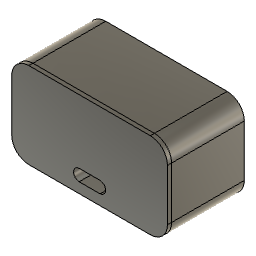
LD2410B Enclosure (Autodesk Fusion 360 design; units mm, degrees)
Autodesk Fusion 360 part; units mm, degrees
sketch "Sketch1" plane through (0, 0, 0) normal (0, 1, 0) x (1, 0, 0)
  line L0 (0, 25.4245) -> (0, -84.4349) construction
  line L1 (0, -3) -> (-3.0467, -3)
  line L2 (-2.98, -4.7) -> (1.5261, -4.7) construction
  arc A0 (-3.0467, -3) -> (-2.98, -6.4013) centre (-2.98, -4.7) ccw
  line L3 (-2.98, -6.4013) -> (0, -6.4013)
  line L4 (2.98, -6.4013) -> (0, -6.4013)
  arc A1 (2.98, -6.4013) -> (3.0467, -3) centre (2.98, -4.7) ccw
  line L5 (0, -3) -> (3.0467, -3)
  line L6 (0, 0) -> (-17.7, 0)
  line L7 (-22.7, -5) -> (-22.7, -20)
  line L8 (-17.7, -25) -> (0, -25)
  line L9 (0, -20) -> (-17.7, -20)
  line L10 (-17.7, -20) -> (-17.7, -12.6)
  line L11 (-17.7, -12.6) -> (0, -12.6)
  line L12 (17.7, -25) -> (0, -25)
  line L13 (0, -20) -> (17.7, -20)
  line L14 (17.7, -20) -> (17.7, -12.6)
  line L15 (22.7, -5) -> (22.7, -20)
  line L16 (17.7, -12.6) -> (0, -12.6)
  line L17 (0, 0) -> (17.7, 0)
  line L18 (17.7, -23.8) -> (-17.7, -23.8)
  line L19 (-21.5, -20) -> (-21.5, -5)
  line L20 (-17.7, -1.2) -> (17.7, -1.2)
  line L21 (21.5, -5) -> (21.5, -20)
  line L22 (-17.7, -20) -> (-17.7, -22)
  line L23 (-17.7, -22) -> (17.7, -22)
  line L24 (17.7, -22) -> (17.7, -20)
  line L25 (17.7, -12.6) -> (17.7, -10.6)
  line L26 (17.7, -10.6) -> (-17.7, -10.6)
  line L27 (-17.7, -10.6) -> (-17.7, -12.6)
  circle A2 centre (-18.3, -9.2) radius 3
  circle A3 centre (-18.3, -9.2) radius 1.4
  circle A4 centre (18.3, -9.2) radius 1.4
  circle A5 centre (18.3, -9.2) radius 3
  arc A6 (17.7, -23.8) -> (21.5, -20) centre (17.7, -20) ccw
  arc A7 (17.7, -25) -> (22.7, -20) centre (17.7, -20) ccw
  arc A8 (21.5, -5) -> (17.7, -1.2) centre (17.7, -5) ccw
  arc A9 (22.7, -5) -> (17.7, 0) centre (17.7, -5) ccw
  arc A10 (-21.5, -20) -> (-17.7, -23.8) centre (-17.7, -20) ccw
  arc A11 (-22.7, -20) -> (-17.7, -25) centre (-17.7, -20) ccw
  arc A12 (-17.7, -1.2) -> (-21.5, -5) centre (-17.7, -5) ccw
  arc A13 (-17.7, 0) -> (-22.7, -5) centre (-17.7, -5) ccw
  point P0 (-22.7, 0)
  point P1 (-22.7, -25)
  dimension "d2" = 1.7
  dimension "d3" = 3
  dimension "d4" = 7.4
  dimension "d5" = 17.7
  dimension "d6" = 5
  dimension "d7" = 25
  dimension "d8" = 5
  dimension "d10" = 1.2
  dimension "d12" = 1.2
  dimension "d13" = 1.2
  dimension "d14" = 1.2
  dimension "d15" = 2
  dimension "d16" = 2
  dimension "d28" = 6
  dimension "d29" = 3.2
  dimension "d30" = 2.8
  dimension "d31" = 8
  dimension "d61" = 3.8
  dimension "d62" = 5
  dimension "d63" = 3.8
  dimension "d64" = 5
  dimension "d65" = 3.8
  dimension "d66" = 5
  dimension "d67" = 3.8
  dimension "d68" = 5
  dimension "d71" = 2.98
  constraint coincident L0 L1.start
  constraint perpendicular L0 L1
  constraint parallel L1 L2
  constraint coincident L2.start A0.centre
  constraint coincident L0 L3.end
  constraint tangent A0 L3
  constraint perpendicular L0 L3
  constraint coincident L6.start L0
  constraint symmetric L0 L1.start L5.start
  constraint symmetric L0 L1.end A1.end
  constraint symmetric L0 A0.end L4.start
  constraint symmetric L0 A0 A1
  constraint symmetric L0 L3.end L4.end
  constraint coincident L6.start L17.start
  constraint perpendicular L0 L6
  constraint perpendicular L6 L7
  constraint coincident L0 L8.end
  constraint perpendicular L0 L8
  constraint coincident L0 L9.start
  constraint perpendicular L0 L9
  constraint perpendicular L9 L10
  constraint coincident L0 L11.end
  constraint perpendicular L0 L11
  constraint symmetric L0 L6.start L17.start
  constraint symmetric L0 L8.end L12.end
  constraint symmetric L0 L9.start L13.start
  constraint symmetric L0 L9.end L13.end
  constraint symmetric L0 L10.end L14.end
  constraint symmetric L0 L11.end L16.end
  constraint perpendicular L0 L18
  constraint perpendicular L18 L19
  constraint perpendicular L15 L20
  constraint perpendicular L18 L21
  constraint perpendicular L9 L22
  constraint perpendicular L14 L23
  constraint perpendicular L13 L24
  constraint perpendicular L16 L25
  constraint perpendicular L10 L26
  constraint perpendicular L11 L27
  constraint concentric A2 A3
  constraint symmetric L0 A2 A5
  constraint symmetric L0 A3 A4
  constraint tangent L21 A6
  constraint tangent L18 A6
  constraint tangent L12 A7
  constraint tangent L15 A7
  constraint tangent L21 A8
  constraint tangent L20 A8
  constraint tangent L15 A9
  constraint tangent L17 A9
  constraint tangent L18 A10
  constraint tangent L19 A10
  constraint coincident P1 L8
  constraint coincident P1 L7
  constraint tangent L8 A11
  constraint tangent L7 A11
  constraint tangent L20 A12
  constraint tangent L19 A12
  constraint coincident P0 L6
  constraint coincident P0 L7
  constraint tangent L6 A13
  constraint tangent L7 A13
  measures "d2" distance of L1 L2
  measures "d3" distance of L5 L6
  measures "d4" distance of L9.end L10.end
  measures "d5" distance of L9.start L9.end
  measures "d6" distance of L8 L9
  measures "d7" distance of P0 P1
  measures "d8" distance of L7 L10
  measures "d10" distance of L12 L18
  measures "d12" distance of L15 L21
  measures "d13" distance of L17 L20
  measures "d14" distance of L7 L19
  measures "d16" distance of L14.end L25.end
  measures "d28" diameter of A2
  measures "d29" distance of L19 A2.centre
  measures "d30" diameter of A3
  measures "d31" distance of L20 A2.centre
  measures "d61" radius of A6
  measures "d62" radius of A7
  measures "d63" radius of A8
  measures "d64" radius of A9
  measures "d65" radius of A10
  measures "d66" radius of A11
  measures "d67" radius of A12
  measures "d68" radius of A13
  measures "d71" distance of L0 L2.start
extrude "Extrude1" add sketch "Sketch1" along normal blind 1.2 contours L1 A0 L3 L4 A1 L5 | L6 L7 L8 L12 L15 L17 A7 A9 A11 A13 | L9 L13 L22 L23 L24 | L9 L10 L11 L13 L14 L16 | L11 L16 L25 L26 L27 A2 A5 | L26 L27 A2 | L26 L27 A2 | L25 L26 A5 | L25 L26 A5 | L18 L19 L20 L21 A6 A8 A10 A12 | A3 | A4 makes body 1
extrude "Extrude2" add sketch "Sketch1" against normal blind 3 contours L9 L13 L22 L23 L24 | L11 L16 L25 L26 L27 A2 A5 | L26 L27 A2 | L25 L26 A5 picked at (-17.2824, -11.486) picked at (17.2824, -11.486) bodies 1
extrude "Extrude3" add sketch "Sketch1" against normal blind 20 contours L6 L7 L8 L12 L15 L17 A7 A9 A11 A13 bodies 1
sketch "Sketch2" plane through (0, -20, 0) normal (0, -1, 0) x (1, 0, 0)
  line L0 (17.7, 1.2) -> (-17.7, 1.2)
  line L1 (-21.5, 5) -> (-21.5, 20)
  line L2 (-17.7, 23.8) -> (17.7, 23.8)
  line L3 (21.5, 20) -> (21.5, 5)
  line L4 (-22.7, 20) -> (-22.7, 5)
  line L5 (-17.7, 0) -> (17.7, 0)
  line L6 (22.7, 5) -> (22.7, 20)
  line L7 (17.7, 25) -> (-17.7, 25)
  line L8 (-2.98, 6.4013) -> (0, 6.4013)
  arc A0 (-2.98, 6.4013) -> (-3.0467, 3) centre (-2.98, 4.7) ccw
  line L9 (0, 3) -> (-3.0467, 3)
  line L10 (0, 3) -> (3.0467, 3)
  arc A1 (3.0467, 3) -> (2.98, 6.4013) centre (2.98, 4.7) ccw
  line L11 (2.98, 6.4013) -> (0, 6.4013)
  line L12 (2.98, 7.6013) -> (0, 7.6013)
  line L13 (-2.98, 7.6013) -> (0, 7.6013)
  arc A2 (-2.98, 7.6013) -> (-3.0672, 1.8) centre (-2.98, 4.7) ccw
  line L14 (0, 1.8) -> (-3.0672, 1.8)
  line L15 (0, 1.8) -> (3.0672, 1.8)
  arc A3 (3.0672, 1.8) -> (2.98, 7.6013) centre (2.98, 4.7) ccw
  line L16 (-17.7, 25) -> (0, 25)
  line L17 (17.7, 25) -> (0, 25)
  line L18 (22.7, 5) -> (22.7, 20)
  line L19 (0, 0) -> (17.7, 0)
  line L20 (0, 0) -> (-17.7, 0)
  line L21 (-22.7, 5) -> (-22.7, 20)
  line L22 (0, 23.6) -> (-17.5, 23.6)
  line L23 (-17.5, 23.6) -> (-17.5, 22.4)
  line L24 (-17.5, 22.4) -> (0, 22.4)
  line L25 (-21.3, 19.8) -> (-20.1, 19.8)
  line L26 (-20.1, 19.8) -> (-20.1, 5.2)
  line L27 (-21.3, 19.8) -> (-21.3, 5.2)
  line L28 (-21.3, 5.2) -> (-20.1, 5.2)
  line L29 (-17.5, 1.4) -> (-17.5, 2.6)
  line L30 (-17.5, 2.6) -> (-7.5, 2.6)
  line L31 (-7.5, 2.6) -> (-7.5, 1.4)
  line L32 (-7.5, 1.4) -> (-17.5, 1.4)
  line L33 (0, -25.4245) -> (0, 84.4349)
  line L34 (0, 23.6) -> (17.5, 23.6)
  line L35 (17.5, 22.4) -> (0, 22.4)
  line L36 (17.5, 23.6) -> (17.5, 22.4)
  line L37 (21.3, 19.8) -> (20.1, 19.8)
  line L38 (20.1, 19.8) -> (20.1, 5.2)
  line L39 (21.3, 19.8) -> (21.3, 5.2)
  line L40 (21.3, 5.2) -> (20.1, 5.2)
  line L41 (17.5, 1.4) -> (17.5, 2.6)
  line L42 (17.5, 2.6) -> (7.5, 2.6)
  line L43 (7.5, 1.4) -> (17.5, 1.4)
  line L44 (7.5, 2.6) -> (7.5, 1.4)
  arc A4 (17.7, 1.2) -> (21.5, 5) centre (17.7, 5) ccw
  arc A5 (-21.5, 5) -> (-17.7, 1.2) centre (-17.7, 5) ccw
  arc A6 (-17.7, 23.8) -> (-21.5, 20) centre (-17.7, 20) ccw
  arc A7 (21.5, 20) -> (17.7, 23.8) centre (17.7, 20) ccw
  arc A8 (17.7, 0) -> (22.7, 5) centre (17.7, 5) ccw
  arc A9 (22.7, 20) -> (17.7, 25) centre (17.7, 20) ccw
  arc A10 (-17.7, 25) -> (-22.7, 20) centre (-17.7, 20) ccw
  arc A11 (-22.7, 5) -> (-17.7, 0) centre (-17.7, 5) ccw
  dimension "d23" = 1.2
  dimension "d34" = 1.2
  dimension "d35" = 1.2
  dimension "d36" = 1.2
  dimension "d37" = 0.2
  dimension "d38" = 0.2
  dimension "d39" = 0.2
  dimension "d40" = 4
  dimension "d41" = 4
  dimension "d42" = 4
  dimension "d43" = 4
  dimension "d44" = 7.5
  constraint parallel L2 L22
  constraint perpendicular L22 L23
  constraint perpendicular L23 L24
  constraint perpendicular L1 L25
  constraint perpendicular L0 L26
  constraint perpendicular L0 L27
  constraint perpendicular L26 L28
  constraint perpendicular L24 L29
  constraint perpendicular L29 L30
  constraint perpendicular L30 L31
  constraint perpendicular L29 L32
  constraint symmetric L22.start L33 L34.start
  constraint symmetric L22.end L33 L34.end
  constraint symmetric L23.end L33 L35.start
  constraint symmetric L24.end L33 L35.end
  constraint symmetric L25.start L33 L37.start
  constraint symmetric L25.end L33 L37.end
  constraint symmetric L26.end L33 L38.end
  constraint symmetric L27.end L33 L39.end
  constraint symmetric L29.start L33 L41.start
  constraint symmetric L29.end L33 L41.end
  constraint symmetric L30.end L33 L42.end
  constraint symmetric L31.end L33 L43.start
  measures "d34" distance of L25.start L25.end
  measures "d35" distance of L22 L24
  measures "d36" distance of L29.start L29.end
  measures "d37" distance of L2 L22
  measures "d38" distance of L1 L27
  measures "d39" distance of L0 L32
  measures "d40" distance of L1 L23
  measures "d41" distance of L2 L25
  measures "d42" distance of L0 L28
  measures "d43" distance of L1 L29.end
  measures "d44" distance of L31 L33
extrude "Extrude4" add sketch "Sketch2" along normal blind 1.2 separate body contours L0 L2 L3 L5 L6 L7 L17 L18 L19 L33 A4 A7 A8 A9 | L0 L2 L3 L12 L15 A3 L33 L34 L35 L36 A4 A7 | L0 L1 L2 L4 L5 L7 L16 L20 L21 L33 A5 A6 A10 A11 | L0 L1 L2 L13 A2 L14 L22 L23 L24 L33 A5 A6 | L10 A1 L11 L12 L15 A3 L33 | L8 A0 L9 L13 A2 L14 L33 | L22 L23 L24 L33 | L33 L34 L35 L36 | L25 L26 L27 L28 | L29 L30 L31 L32 | L37 L38 L39 L40 | L41 L42 L43 L44 makes body 2
extrude "Extrude5" add sketch "Sketch2" against normal blind 8 contours L10 A1 L11 L12 L15 A3 L33 | L8 A0 L9 L13 A2 L14 L33 bodies 2
extrude "Extrude7" add sketch "Sketch2" against normal blind 2.5 contours L22 L23 L24 L33 | L33 L34 L35 L36 | L25 L26 L27 L28 | L29 L30 L31 L32 | L37 L38 L39 L40 | L41 L42 L43 L44 bodies 2
sketch "Sketch4" plane through (17.5, 0, 0) normal (1, 0, 0) x (0, 1, 0)
  line L0 (-20, 23.6) -> (-20, 22.4)
  line L1 (-20, 22.4) -> (-17.5, 22.4)
  line L2 (-17.5, 22.4) -> (-17.5, 23.6)
  line L3 (-17.5, 23.6) -> (-20, 23.6)
  line L4 (-19, 24.1) -> (-18.5, 23.6)
  line L5 (-19, 24.1) -> (-17.815, 24.1) construction
  line L6 (-19, 24.1) -> (-19.5, 23.6)
  line L7 (-18.5, 23.6) -> (-19.5, 23.6)
  line L8 (-17.5, 5.2) -> (-17.5, 19.8) construction
  line L9 (-17.5, 12.5) -> (-15.1425, 12.5) construction
  line L10 (-18.5, 1.4) -> (-19.5, 1.4)
  line L11 (-19, 0.9) -> (-19.5, 1.4)
  line L12 (-19, 0.9) -> (-18.5, 1.4)
  line L13 (-18.2586, 23.5) -> (-19.7414, 23.5)
  line L14 (-19, 24.2414) -> (-19.7414, 23.5)
  line L15 (-19, 24.2414) -> (-18.2586, 23.5)
  line L16 (-19, 0.7586) -> (-19.7414, 1.5)
  line L17 (-19, 0.7586) -> (-18.2586, 1.5)
  line L18 (-18.2586, 1.5) -> (-19.7414, 1.5)
  dimension "d47" = 45
  dimension "d48" = 0.5
  dimension "d49" = 1
  dimension "d57" = 0.1
  constraint horizontal L5
  constraint coincident L3 L4.end
  constraint coincident L3 L6.end
  constraint perpendicular L4 L6
  constraint midpoint L8 L9.start
  constraint perpendicular L8 L9
  constraint symmetric L4.start L9 L11.start
  constraint symmetric L4.end L9 L10.start
  constraint symmetric L6.end L9 L10.end
  constraint symmetric L9 L13.start L17.end
  constraint symmetric L9 L13.end L16.end
  constraint symmetric L9 L14.start L16.start
  measures "d47" angle of L4 L5
  measures "d48" distance of L3 L4.start
  measures "d49" distance of L2 L4.end
extrude "Extrude8" add sketch "Sketch4" against normal up to surface (35 mm away) contours L3 L4 L6 L7 bodies 2
extrude "Extrude9" add sketch "Sketch4" against normal up to surface (10 mm away) contours L10 L11 L12 bodies 2
extrude "Extrude10" add sketch "Sketch4" against normal up to surface (9 mm away) from surface at -26 contours L10 L11 L12 bodies 2
extrude "Extrude11" cut sketch "Sketch4" against normal blind 35.6 from surface at 0.3 contours L3 L4 L6 L14 L15 | L10 L11 L12 bodies 1
sketch "Sketch5" plane through (0, 1.2, 0) normal (0, 1, 0) x (-1, 0, 0)
  line L0 (-17.7, 0) -> (17.7, 0)
  arc A0 (17.7, 0) -> (22.7, 5) centre (17.7, 5) ccw
  line L1 (22.7, 5) -> (22.7, 20)
  arc A1 (22.7, 20) -> (17.7, 25) centre (17.7, 20) ccw
  line L2 (17.7, 25) -> (-17.7, 25)
  arc A2 (-17.7, 25) -> (-22.7, 20) centre (-17.7, 20) ccw
  line L3 (-22.7, 20) -> (-22.7, 5)
  arc A3 (-22.7, 5) -> (-17.7, 0) centre (-17.7, 5) ccw
  line L4 (22.7, 12.5) -> (-22.7, 12.5) construction
  line L5 (0, 25) -> (0, 0) construction
  spline S0 degree 2 poles (0.0295, 1.603) (-2.2457, 1.603) (-4.2468, 2.4665) knots 0 0 0 1 1 1
  spline S1 degree 2 poles (-4.2468, 2.4665) (-6.2478, 3.33) (-7.7281, 4.8102) knots 0 0 0 1 1 1
  spline S2 degree 2 poles (-7.7281, 4.8102) (-9.2083, 6.2905) (-10.0718, 8.2915) knots 0 0 0 1 1 1
  spline S3 degree 2 poles (-10.0718, 8.2915) (-10.9353, 10.2926) (-10.9353, 12.5678) knots 0 0 0 1 1 1
  spline S4 degree 2 poles (-10.9353, 12.5678) (-10.9353, 14.843) (-10.0718, 16.8441) knots 0 0 0 1 1 1
  spline S5 degree 2 poles (-10.0718, 16.8441) (-9.2083, 18.8451) (-7.7281, 20.3254) knots 0 0 0 1 1 1
  spline S6 degree 2 poles (-7.7281, 20.3254) (-6.2478, 21.8056) (-4.2468, 22.6691) knots 0 0 0 1 1 1
  spline S7 degree 2 poles (-4.2468, 22.6691) (-2.2457, 23.5326) (0.0295, 23.5326) knots 0 0 0 1 1 1
  spline S8 degree 2 poles (0.0295, 23.5326) (2.3047, 23.5326) (4.3058, 22.6691) knots 0 0 0 1 1 1
  spline S9 degree 2 poles (4.3058, 22.6691) (6.3068, 21.8056) (7.7871, 20.3254) knots 0 0 0 1 1 1
  spline S10 degree 2 poles (7.7871, 20.3254) (9.2673, 18.8451) (10.1308, 16.8441) knots 0 0 0 1 1 1
  spline S11 degree 2 poles (10.1308, 16.8441) (10.9943, 14.843) (10.9943, 12.5678) knots 0 0 0 1 1 1
  spline S12 degree 2 poles (10.9943, 12.5678) (10.9943, 10.2926) (10.1308, 8.2915) knots 0 0 0 1 1 1
  spline S13 degree 2 poles (10.1308, 8.2915) (9.2673, 6.2905) (7.7871, 4.8102) knots 0 0 0 1 1 1
  spline S14 degree 2 poles (7.7871, 4.8102) (6.3068, 3.33) (4.3058, 2.4665) knots 0 0 0 1 1 1
  spline S15 degree 2 poles (4.3058, 2.4665) (2.3047, 1.603) (0.0295, 1.603) knots 0 0 0 1 1 1
  spline S16 degree 2 poles (0.0295, 3.2477) (1.7565, 3.2477) (3.2778, 3.8097) knots 0 0 0 1 1 1
  spline S17 degree 2 poles (3.2778, 3.8097) (4.7992, 4.3716) (6.0327, 5.4133) knots 0 0 0 1 1 1
  line L6 (6.0327, 5.4133) -> (4.0591, 7.3595)
  spline S18 degree 2 poles (4.0591, 7.3595) (3.2093, 6.729) (2.1951, 6.359) knots 0 0 0 1 1 1
  spline S19 degree 2 poles (2.1951, 6.359) (1.1808, 5.9889) (0.0295, 5.9889) knots 0 0 0 1 1 1
  spline S20 degree 2 poles (0.0295, 5.9889) (-2.7117, 5.9889) (-4.6305, 7.9078) knots 0 0 0 1 1 1
  spline S21 degree 2 poles (-4.6305, 7.9078) (-6.5494, 9.8266) (-6.5494, 12.5678) knots 0 0 0 1 1 1
  spline S22 degree 2 poles (-6.5494, 12.5678) (-6.5494, 15.309) (-4.6305, 17.2278) knots 0 0 0 1 1 1
  spline S23 degree 2 poles (-4.6305, 17.2278) (-2.7117, 19.1467) (0.0295, 19.1467) knots 0 0 0 1 1 1
  spline S24 degree 2 poles (0.0295, 19.1467) (2.7707, 19.1467) (4.6895, 17.2278) knots 0 0 0 1 1 1
  spline S25 degree 2 poles (4.6895, 17.2278) (6.6084, 15.309) (6.6084, 12.5678) knots 0 0 0 1 1 1
  spline S26 degree 2 poles (6.6084, 12.5678) (6.6084, 11.4165) (6.2383, 10.4022) knots 0 0 0 1 1 1
  spline S27 degree 2 poles (6.2383, 10.4022) (5.8683, 9.388) (5.2378, 8.5382) knots 0 0 0 1 1 1
  line L7 (5.2378, 8.5382) -> (7.184, 6.592)
  spline S28 degree 2 poles (7.184, 6.592) (8.1983, 7.8255) (8.7739, 9.3332) knots 0 0 0 1 1 1
  spline S29 degree 2 poles (8.7739, 9.3332) (9.3496, 10.8408) (9.3496, 12.5678) knots 0 0 0 1 1 1
  spline S30 degree 2 poles (9.3496, 12.5678) (9.3496, 16.4603) (6.6358, 19.1741) knots 0 0 0 1 1 1
  spline S31 degree 2 poles (6.6358, 19.1741) (3.922, 21.8879) (0.0295, 21.8879) knots 0 0 0 1 1 1
  spline S32 degree 2 poles (0.0295, 21.8879) (-3.863, 21.8879) (-6.5768, 19.1741) knots 0 0 0 1 1 1
  spline S33 degree 2 poles (-6.5768, 19.1741) (-9.2905, 16.4603) (-9.2905, 12.5678) knots 0 0 0 1 1 1
  spline S34 degree 2 poles (-9.2905, 12.5678) (-9.2905, 8.6753) (-6.5768, 5.9615) knots 0 0 0 1 1 1
  spline S35 degree 2 poles (-6.5768, 5.9615) (-3.863, 3.2477) (0.0295, 3.2477) knots 0 0 0 1 1 1
  spline S36 degree 2 poles (0.0295, 7.6336) (0.8245, 7.6336) (1.5509, 7.8666) knots 0 0 0 1 1 1
  spline S37 degree 2 poles (1.5509, 7.8666) (2.2773, 8.0996) (2.8804, 8.5382) knots 0 0 0 1 1 1
  line L8 (2.8804, 8.5382) -> (0.8519, 10.5393)
  spline S38 degree 2 poles (0.8519, 10.5393) (0.66, 10.4571) (0.4544, 10.4159) knots 0 0 0 1 1 1
  spline S39 degree 2 poles (0.4544, 10.4159) (0.2488, 10.3748) (0.0295, 10.3748) knots 0 0 0 1 1 1
  spline S40 degree 2 poles (0.0295, 10.3748) (-0.8751, 10.3748) (-1.5193, 11.019) knots 0 0 0 1 1 1
  spline S41 degree 2 poles (-1.5193, 11.019) (-2.1634, 11.6632) (-2.1634, 12.5678) knots 0 0 0 1 1 1
  spline S42 degree 2 poles (-2.1634, 12.5678) (-2.1634, 13.4724) (-1.5193, 14.1166) knots 0 0 0 1 1 1
  spline S43 degree 2 poles (-1.5193, 14.1166) (-0.8751, 14.7607) (0.0295, 14.7607) knots 0 0 0 1 1 1
  spline S44 degree 2 poles (0.0295, 14.7607) (0.9341, 14.7607) (1.5783, 14.1166) knots 0 0 0 1 1 1
  spline S45 degree 2 poles (1.5783, 14.1166) (2.2225, 13.4724) (2.2225, 12.5678) knots 0 0 0 1 1 1
  spline S46 degree 2 poles (2.2225, 12.5678) (2.2225, 12.3485) (2.1676, 12.1292) knots 0 0 0 1 1 1
  spline S47 degree 2 poles (2.1676, 12.1292) (2.1128, 11.9099) (2.0306, 11.6906) knots 0 0 0 1 1 1
  line L9 (2.0306, 11.6906) -> (4.0591, 9.7169)
  spline S48 degree 2 poles (4.0591, 9.7169) (4.4977, 10.32) (4.7307, 11.0464) knots 0 0 0 1 1 1
  spline S49 degree 2 poles (4.7307, 11.0464) (4.9637, 11.7728) (4.9637, 12.5678) knots 0 0 0 1 1 1
  spline S50 degree 2 poles (4.9637, 12.5678) (4.9637, 14.6237) (3.5245, 16.0628) knots 0 0 0 1 1 1
  spline S51 degree 2 poles (3.5245, 16.0628) (2.0854, 17.5019) (0.0295, 17.5019) knots 0 0 0 1 1 1
  spline S52 degree 2 poles (0.0295, 17.5019) (-2.0264, 17.5019) (-3.4655, 16.0628) knots 0 0 0 1 1 1
  spline S53 degree 2 poles (-3.4655, 16.0628) (-4.9046, 14.6237) (-4.9046, 12.5678) knots 0 0 0 1 1 1
  spline S54 degree 2 poles (-4.9046, 12.5678) (-4.9046, 10.5119) (-3.4655, 9.0728) knots 0 0 0 1 1 1
  spline S55 degree 2 poles (-3.4655, 9.0728) (-2.0264, 7.6336) (0.0295, 7.6336) knots 0 0 0 1 1 1
  constraint midpoint L1 L4.start
  constraint midpoint L3 L4.end
  constraint midpoint L2 L5.start
  constraint coincident L5.end origin
extrude "Extrude12" cut sketch "Sketch5" against normal blind 0.2 contours S0 S1 S2 S3 S4 S5 S6 S7 S8 S9 S10 S11 S12 S13 S14 S15 bodies 1
equation "d5 = ( 35.4 / 2 ) * 1 mm"
